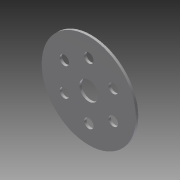
# Autodesk Inventor part: Plate (Front)
Saved by Autodesk Inventor 2014 (Build 180170000, 170)
## iProperties
Created: 2014-01-12
Part Number: Plate (Front)
Material: Steel
Document SubType Name: Sheet Metal
Designer: Andrew Toennies
Mass: 82.0888 g
Surface Area: 83.6067 cm^2
Volume: 10.4572 cm^3
Density: 7.85 g/cm^3
Sheet Metal Rule: Default
Appearance: Steel
Author: Andrew Toennies
Autodesk Inventor part; units mm, degrees
ref_plane "YZ Plane" through (0, 0, 0) normal (1, 0, 0) x (0, 1, 0)
ref_plane "XZ Plane" through (0, 0, 0) normal (0, 1, 0) x (-1, 0, 0)
ref_plane "XY Plane" through (0, 0, 0) normal (0, 0, 1) x (1, 0, 0)
sketch "Sketch1" plane through (0, 0, 0) normal (0, 0, 1) x (1, 0, 0)
  circle A0 centre (0, 0) radius 63.5
  circle A1 centre (0, 0) radius 12.7
  circle A2 centre (0, 41.275) radius 6.35
  line L0 (0, 0) -> (0, 41.275) construction
  circle A3 centre (0, 41.275) radius 16.6687 construction
  circle A4 centre (0, 57.9438) radius 2.3812
  circle A5 centre (16.6688, 41.275) radius 2.3812
  circle A6 centre (0, 24.6063) radius 2.3812
  circle A7 centre (-16.6688, 41.275) radius 2.3813
  line L1 (0, 41.275) -> (0, 57.9438) construction
  line L2 (-16.6688, 41.275) -> (16.6688, 41.275) construction
  circle A8 centre (-35.7452, 20.6375) radius 6.35
  circle A9 centre (-50.1808, 28.9719) radius 2.3812
  circle A10 centre (-27.4108, 35.0731) radius 2.3812
  circle A11 centre (-21.3096, 12.3031) radius 2.3812
  circle A12 centre (-44.0796, 6.2019) radius 2.3813
  circle A13 centre (-35.7452, -20.6375) radius 6.35
  circle A14 centre (-50.1808, -28.9719) radius 2.3812
  circle A15 centre (-44.0796, -6.2019) radius 2.3812
  circle A16 centre (-21.3096, -12.3031) radius 2.3812
  circle A17 centre (-27.4108, -35.0731) radius 2.3813
  circle A18 centre (0, -41.275) radius 6.35
  circle A19 centre (0, -57.9438) radius 2.3812
  circle A20 centre (-16.6688, -41.275) radius 2.3812
  circle A21 centre (0, -24.6062) radius 2.3812
  circle A22 centre (16.6687, -41.275) radius 2.3813
  circle A23 centre (35.7452, -20.6375) radius 6.35
  circle A24 centre (50.1808, -28.9719) radius 2.3812
  circle A25 centre (27.4108, -35.0731) radius 2.3812
  circle A26 centre (21.3096, -12.3031) radius 2.3812
  circle A27 centre (44.0796, -6.2019) radius 2.3813
  circle A28 centre (35.7452, 20.6375) radius 6.35
  circle A29 centre (50.1808, 28.9719) radius 2.3812
  circle A30 centre (44.0796, 6.2019) radius 2.3812
  circle A31 centre (21.3096, 12.3031) radius 2.3812
  circle A32 centre (27.4108, 35.0731) radius 2.3813
  dimension "d0" = 127
  dimension "d1" = 25.4
  dimension "d2" = 12.7
  dimension "d3" = 41.275
  dimension "d9" = 33.3375
  dimension "d11" = 4.7625
  dimension "d12" = 4.7625
  dimension "d13" = 4.7625
  dimension "d14" = 4.7625
  dimension "d17" = 360
  measures "d0" diameter of A0
  measures "d1" diameter of A1
  measures "d2" diameter of A2
  measures "d3" distance of L0.start L0.end
  measures "d9" diameter of A3
  measures "d11" diameter of A4
  measures "d12" diameter of A5
  measures "d13" diameter of A6
  measures "d14" diameter of A7
extrude "Plate2" add sketch "Sketch1" along normal blind 3.175
equation "\"BendRadius\" = Thickness"
equation "\"BendReliefWidth\" = Thickness"
equation "\"BendReliefDepth\" = 0.5 * Thickness"
equation "\"CornerReliefSize\" = 4 * Thickness"
equation "\"MinimumRemnant\" = 2 * Thickness"
equation "\"TransitionRadius\" = BendRadius"
equation "\"JacobiRadiusSize\" = BendRadius"
equation "\"GapSize\" = Thickness"
equation "\"d8\" = BendRadius"
equation "\"d19\" = BendRadius"
equation "\"Thickness\" = 3.175"
body "Solid2"
